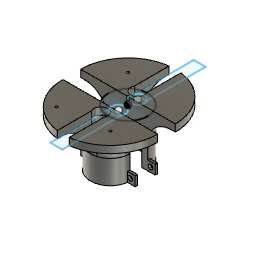
Tennis nozzle connector for ViveTracker (Autodesk Fusion 360 design; units mm, degrees)
Autodesk Fusion 360 part; units mm, degrees
note: some values were not read from the file. Set by a fixed rule: which sketch regions a step uses.
sketch "Sketch1" plane through (0, 0, 0) normal (0, 0, 1) x (1, 0, 0)
  circle A0 centre (0, 0) radius 11.65
  circle A1 centre (0, 0) radius 16.65
  dimension "d1" = 23.3
  dimension "d2" = 33.3
  constraint coincident A0.centre A1.centre
  measures "d1" diameter of A0
  measures "d2" diameter of A1
sketch "Sketch6" plane through (0, 0, 0) normal (0, 0, 1) x (1, 0, 0)
  circle A0 centre (0, 0) radius 40
  dimension "d39" = 80
  constraint coincident A0.centre origin
  measures "d39" diameter of A0
extrude "Extrude6" add sketch "Sketch6" along normal blind 6 makes body 1
extrude "Extrude1" add sketch "Sketch1" along normal blind 20 separate body makes body 2
sketch "Sketch7" plane through (0, 0, 6) normal (0, 0, 1) x (-1, 0, 0)
  circle A0 centre (0, 0) radius 40
  circle A1 centre (0, 0) radius 1
  circle A2 centre (-25, 0) radius 1
  circle A3 centre (25, 0) radius 1
  circle A4 centre (0, 32) radius 1
  dimension "d42" = 2
  dimension "d44" = 2
  dimension "d45" = 2
  dimension "d46" = 2
  constraint coincident A0.centre A1.centre
  measures "d42" diameter of A1
  measures "d44" diameter of A2
  measures "d45" diameter of A3
  measures "d46" diameter of A4
extrude "Extrude7" cut sketch "Sketch7" against normal blind 3 contours A1 | A2 | A3 | A4 bodies 1
ref_plane "WorkPlane1" through (0, 0, 20) normal (0, 0, 1) x (1, 0, 0)
ref_plane "WorkPlane2" through (0, 0, 40) normal (0, 0, 1) x (1, 0, 0)
sketch "Sketch4" plane through (0, 0, 40) normal (0, 0, 1) x (1, 0, 0)
  circle A0 centre (0, 0) radius 16.65
  circle A1 centre (0, 8) radius 5.65
  circle A2 centre (0, -8) radius 5.65
  line L0 (-5, -10.5) -> (5, -10.5)
  line L1 (5, -10.5) -> (5, -60.5)
  line L2 (5, -60.5) -> (-5, -60.5)
  line L3 (-5, -60.5) -> (-5, -10.5)
  line L4 (-5, 60.5) -> (5, 60.5)
  line L5 (-5, 10.5) -> (-5, 60.5)
  line L6 (5, 60.5) -> (5, 10.5)
  line L7 (5, 10.5) -> (-5, 10.5)
  dimension "d27" = 33.3
  dimension "d28" = 11.3
  dimension "d29" = 11.3
  dimension "d30" = 10
  dimension "d31" = 50
  dimension "d32" = 10
  dimension "d33" = 50
  constraint coincident A0.centre origin
  constraint horizontal L0
  constraint vertical L1
  constraint horizontal L2
  constraint vertical L3
  constraint horizontal L4
  constraint vertical L6
  constraint horizontal L7
  constraint vertical L5
  measures "d27" diameter of A0
  measures "d28" diameter of A1
  measures "d29" diameter of A2
  measures "d30" distance of L0.start L0.end
  measures "d31" distance of L0.start L2.end
  measures "d32" distance of L4.start L4.end
  measures "d33" distance of L5.start L4.start
extrude "Extrude4" add sketch "Sketch4" against normal blind 20 contours A0 A1 A2 L1 L3 L5 L6 | A0 A1 L5 L6 | A0 A2 L1 L3 | A1 L5 L6 L7 | A1 L5 L6 L7 | A2 L0 L1 L3 | A2 L0 L1 L3 bodies 2
move_body "Move2" bodies 1 to x (0.707107, -0.707107, 0) y (0.707107, 0.707107, 0) z (0, 0, 1) at (0, 0, 0)
move_body "Move3" bodies 1 to x (1, 0, 0) y (0, 1, 0) z (0, 0, 1) at (0, 0, 40)
extrude "Extrude5" cut sketch "Sketch4" against normal blind 20 draft -0.5 contours A0 A1 L5 L6 | A0 L4 L5 L6 | A0 L1 L2 L3 | A0 A2 L1 L3 | A1 L5 L6 L7 | A1 L5 L6 L7 | A2 L0 L1 L3 | A2 L0 L1 L3 bodies 2
extrude "Extrude8" cut sketch "Sketch4" along normal blind 10 contours A0 A1 L5 L6 | A0 L4 L5 L6 | A0 L1 L2 L3 | A0 A2 L1 L3 | A1 L5 L6 L7 | A1 L5 L6 L7 | A2 L0 L1 L3 | A2 L0 L1 L3 bodies 1
sketch "Sketch3" plane through (0, 0, 0) normal (0, 1, 0) x (1, 0, 0)
  line L0 (15, -8) -> (23, -8)
  line L1 (23, -8) -> (23, 0)
  line L2 (23, 0) -> (15, 0)
  line L3 (15, 0) -> (15, -8)
  circle A0 centre (19, -4) radius 2
  circle A1 centre (-19, -4) radius 2
  line L4 (-23, -8) -> (-15, -8)
  line L5 (-15, -8) -> (-15, 0)
  line L6 (-15, 0) -> (-23, 0)
  line L7 (-23, 0) -> (-23, -8)
  dimension "d16" = 8
  dimension "d17" = 8
  dimension "d18" = 4
  dimension "d19" = 8
  dimension "d20" = 8
  dimension "d21" = 4
  constraint horizontal L0
  constraint vertical L1
  constraint horizontal L2
  constraint vertical L3
  constraint horizontal L4
  constraint vertical L5
  constraint horizontal L6
  constraint vertical L7
  measures "d16" distance of L0.start L0.end
  measures "d17" distance of L0.start L2.end
  measures "d18" diameter of A0
  measures "d19" distance of L4.end L4.start
  measures "d20" distance of L6.end L4.start
  measures "d21" diameter of A1
extrude "Extrude3" add sketch "Sketch3" along normal blind 2 and the other way blind 2 bodies 2
combine "Combine1" operation add target body 1 tool bodies 2
fillet "Fillet2" radius 20 2 edges at (-16.65, 0, 40) (16.65, 0, 40) on bodies 1
split "Split1" by plane through (0, 0, 0) normal (0, 1, 0) bodies 1 makes body 3 at (-21.0495, 7.5101, 46)
move_body "Move1" bodies 1 to x (1, 0, 0) y (0, 1, 0) z (0, 0, 1) at (0, -15, 0)
fillet "Fillet1" [suppressed]
